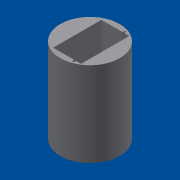
# Autodesk Inventor part: Zack-Zack
Saved by Autodesk Inventor 2015 (Build 190159000, 159)
## iProperties
Created: 2018-02-27
Part Number: Zack-Zack
Material: Generisch
Document SubType Name: Modeling
Designer: Florian Schwanse
Density: 1 g/cm^3
Appearance: Vorgabe
Author: Florian Schwanse
Autodesk Inventor part; units mm, degrees
ref_plane "YZ Plane" through (0, 0, 0) normal (1, 0, 0) x (0, 1, 0)
ref_plane "XZ Plane" through (0, 0, 0) normal (0, 1, 0) x (-1, 0, 0)
ref_plane "XY Plane" through (0, 0, 0) normal (0, 0, 1) x (1, 0, 0)
sketch "Skizze1" plane through (0, 0, 0) normal (0, 0, 1) x (1, 0, 0)
  circle A0 centre (0, 0) radius 35
  dimension "d0" = 70
  constraints: 1 centre point, 1 coincident
  measures "d0" diameter of A0
extrude "Extrusion1" add sketch "Skizze1" along normal blind 100
sketch "Skizze2" plane through (0, 0, 100) normal (0, 0, 1) x (1, 0, 0)
  line L0 (10, -31) -> (12, -31)
  line L1 (12, -31) -> (12, 31)
  line L2 (12, 31) -> (10, 31)
  line L3 (10, 31) -> (10, -31)
  point P0 (0, 0)
  point P1 (10, 0)
  dimension "d3" = 2
  dimension "d4" = 62
  dimension "d5" = 10
  constraints: 8 end point, 2 parallel, 1 horizontal, 1 horizontal alignment, 1 midpoint, 1 perpendicular
  measures "d3" distance between parallel lines of L3 L1
  measures "d4" distance between parallel lines of L2 L0
  measures "d5" distance from line of point (0, 0) L3
extrude "Extrusion2" cut sketch "Skizze2" against normal blind 80
sketch "Skizze3" plane through (0, 0, 100) normal (0, 0, 1) x (1, 0, 0)
  line L0 (-15, -28.5) -> (18, -28.5)
  line L1 (18, -28.5) -> (18, 28.5)
  line L2 (18, 28.5) -> (-15, 28.5)
  line L3 (-15, 28.5) -> (-15, -28.5)
  line L4 (10, -31) -> (10, 31) projected
  point P0 (0, 0)
  point P1 (-15, 0)
  dimension "d8" = 8
  dimension "d9" = 57
  dimension "d10" = 25
  constraints: 8 end point, 2 parallel, 1 horizontal, 1 horizontal alignment, 1 midpoint, 1 perpendicular
  measures "d8" distance between parallel lines of L4 L1
  measures "d9" distance between parallel lines of L0 L2
  measures "d10" distance between parallel lines of L3 L4
extrude "Extrusion3" cut sketch "Skizze3" against normal blind 80
sketch "Skizze4" plane through (0, 0, 0) normal (0, 0, -1) x (-1, 0, 0)
  line L0 (-13.5, -13.5) -> (13.5, -13.5)
  line L1 (13.5, -13.5) -> (13.5, 13.5)
  line L2 (13.5, 13.5) -> (-13.5, 13.5)
  line L3 (-13.5, 13.5) -> (-13.5, -13.5)
  line L4 (-13.5, -13.5) -> (13.5, 13.5) construction
  line L5 (13.5, -13.5) -> (-13.5, 13.5) construction
  point P0 (0, 0)
  dimension "d13" = 27
  dimension "d14" = 27
  constraints: 12 end point, 2 midpoint, 2 parallel, 1 horizontal, 1 perpendicular
  measures "d13" distance between parallel lines of L0 L2
  measures "d14" distance between parallel lines of L3 L1
extrude "Extrusion4" cut sketch "Skizze4" against normal blind 4
sketch "Skizze5" plane through (0, 0, 0) normal (0, 0, -1) x (-1, 0, 0)
  line L0 (-11, -11) -> (11, -11)
  line L1 (11, -11) -> (11, 11)
  line L2 (11, 11) -> (-11, 11)
  line L3 (-11, 11) -> (-11, -11)
  line L4 (-11, -11) -> (11, 11) construction
  line L5 (11, -11) -> (-11, 11) construction
  point P0 (0, 0)
  dimension "d17" = 22
  dimension "d18" = 22
  constraints: 12 end point, 2 midpoint, 2 parallel, 1 horizontal, 1 perpendicular
  measures "d17" distance between parallel lines of L3 L1
  measures "d18" distance between parallel lines of L2 L0
extrude "Extrusion5" cut sketch "Skizze5" against normal blind 15
sketch "Skizze6" plane through (0, 0, 0) normal (0, 0, -1) x (-1, 0, 0)
  line L0 (14, 9) -> (8, 9)
  line L1 (8, 9) -> (8, -9)
  line L2 (8, -9) -> (14, -9)
  line L3 (14, -9) -> (14, 9)
  point P0 (0, 0)
  point P1 (8, 0)
  dimension "d22" = 8
  dimension "d23" = 6
  dimension "d24" = 18
  constraints: 8 end point, 2 parallel, 1 horizontal, 1 horizontal alignment, 1 midpoint, 1 perpendicular
  measures "d22" distance from line of L1 point (0, 0)
  measures "d23" distance between parallel lines of L3 L1
  measures "d24" distance between parallel lines of L2 L0
extrude "Extrusion6" cut sketch "Skizze6" against normal through all
equation "\"d13\" = d14"
equation "\"d18\" = d17"
